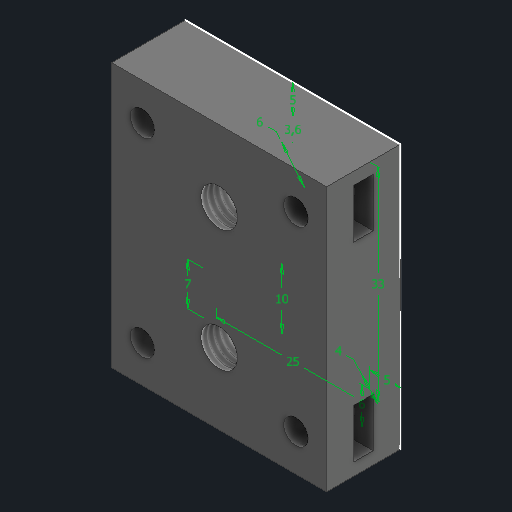
# Autodesk Inventor part: LoadCellBase
Saved by Autodesk Inventor 2027 (Build 310192060, 192F)
## iProperties
Created: 2026-10-06
Part Number: LoadCellBase
Material: Genérico
Document SubType Name: Modeling
Designer: EspacoMaker
Density: 1 g/cm^3
Appearance: Padrão
Author: EspacoMaker
Autodesk Inventor part; units mm, degrees
ref_plane "YZ Plane" through (0, 0, 0) normal (1, 0, 0) x (0, 1, 0)
ref_plane "XZ Plane" through (0, 0, 0) normal (0, 1, 0) x (-1, 0, 0)
ref_plane "XY Plane" through (0, 0, 0) normal (0, 0, 1) x (1, 0, 0)
sketch "EsboçoBase" plane through (0, 0, 0) normal (0, 0, 1) x (1, 0, 0)
  line L0 (-12.5, 16.5) -> (12.5, 16.5) construction
  line L1 (12.5, 16.5) -> (12.5, -16.5) construction
  line L2 (12.5, -16.5) -> (-12.5, -16.5) construction
  line L3 (-12.5, -16.5) -> (-12.5, 16.5) construction
  line L4 (-12.5, 16.5) -> (12.5, -16.5) construction
  line L5 (12.5, 16.5) -> (-12.5, -16.5) construction
  line L6 (0, 16.5) -> (0, -16.5) construction
  line L7 (-12.5, 12.9) -> (12.5, 12.9) construction
  circle A0 centre (0, 9.9) radius 3
  line L8 (-12.5, 0) -> (12.5, 0) construction
  circle A1 centre (0, -9.9) radius 3
  line L9 (17.5, 21.5) -> (-17.5, 21.5)
  line L10 (-17.5, 21.5) -> (-17.5, -21.5)
  line L11 (-17.5, -21.5) -> (17.5, -21.5)
  line L12 (17.5, -21.5) -> (17.5, 21.5)
  line L13 (-2.8868, -4.9) -> (2.8868, -4.9)
  line L14 (2.8868, -4.9) -> (5.7735, -9.9)
  line L15 (5.7735, -9.9) -> (2.8868, -14.9)
  line L16 (2.8868, -14.9) -> (-2.8868, -14.9)
  line L17 (-2.8868, -14.9) -> (-5.7735, -9.9)
  line L18 (-5.7735, -9.9) -> (-2.8868, -4.9)
  line L19 (-2.8868, 4.9) -> (2.8868, 4.9)
  line L20 (2.8868, 4.9) -> (5.7735, 9.9)
  line L21 (5.7735, 9.9) -> (2.8868, 14.9)
  line L22 (2.8868, 14.9) -> (-2.8868, 14.9)
  line L23 (-2.8868, 14.9) -> (-5.7735, 9.9)
  line L24 (-5.7735, 9.9) -> (-2.8868, 4.9)
  circle A2 centre (12.5, -15.5) radius 2
  circle A3 centre (12.5, 15.5) radius 2
  circle A4 centre (-12.5, -15.5) radius 2
  circle A5 centre (-12.5, 15.5) radius 2
  line L25 (-14.5207, -12) -> (-10.4793, -12)
  line L26 (-10.4793, -12) -> (-8.4585, -15.5)
  line L27 (-8.4585, -15.5) -> (-10.4793, -19)
  line L28 (-10.4793, -19) -> (-14.5207, -19)
  line L29 (-14.5207, -19) -> (-16.5415, -15.5)
  line L30 (-16.5415, -15.5) -> (-14.5207, -12)
  point P0 (0, 0)
  point P1 (0, -9.9)
  dimension "d0" = 25
  dimension "d1" = 33
  dimension "d2" = 3.6
  dimension "d3" = 6
  dimension "d4" = 5
  dimension "d22" = 10
  dimension "d29" = 4
  dimension "d30" = 6
  dimension "d31" = 5
  dimension "d38" = 7
  constraints: 62 end point, 10 symmetric about line, 6 centre point, 6 midpoint, 5 parallel, 3 horizontal, 2 coincident, 2 perpendicular, 1 point on line, 1 tangent, 33 other
  measures "d0" distance of L1.end L2.end
  measures "d1" distance of L0.end L1.end
  measures "d2" distance between parallel lines of L0 L7
  measures "d3" diameter of A0
  measures "d4" distance between parallel lines of L0 L9
  measures "d22" distance between parallel lines of L13 L16
  measures "d29" diameter of A2
  measures "d30" distance from line of A2.centre L11
  measures "d31" distance from line of L12 A2.centre
  measures "d38" distance between parallel lines of L25 L28
extrude "Adaptador" add sketch "EsboçoBase" along normal blind 12 contours A0 | A1 | L12 L11 L10 L9 | L13 L14 L15 L16 L17 L18 | L24 L23 L22 L21 L20 L19 | A2 | A3 | A4 | A5 | L25 L26 L27 L28 L29 L30
extrude "Furos" cut sketch "EsboçoBase" along normal blind 15 contours A0 | A1
thread "Thread1" size "M6x1" class "6H" standard "ANSI Metric M Profile" full length
thread "Thread2" size "M6x1" class "6H" standard "ANSI Metric M Profile" full length
sketch "Sketch5" plane through (-17.5, -21.5, 0) normal (-1, 0, 0) x (0, 0, 1)
  point P0 (0, 21.5)
extrude "Extrusion5" cut sketch "EsboçoBase" along normal blind 2 contours L13 L14 L15 L16 L17 L18 | L24 L23 L22 L21 L20 L19
sketch "PorcasLaterais" plane through (-17.5, -21.5, 0) normal (-1, 0, 0) x (0, 0, 1)
  line L0 (4.4, 2) -> (7.6, 2)
  line L1 (7.6, 2) -> (7.6, 10)
  line L2 (7.6, 10) -> (4.4, 10)
  line L3 (4.4, 10) -> (4.4, 2)
  line L4 (0, 0) -> (12, 0) projected
  line L5 (0, 43) -> (0, 0) projected
  line L6 (4.4, 6) -> (7.6, 6) construction
  line L7 (6, 2) -> (6, 10) construction
  line L8 (6, 0) -> (6, 43) construction
  line L9 (0, 6) -> (12, 6) construction
  line L10 (12, 43) -> (12, 0) projected
  point P0 (0, 21.5)
  dimension "d32" = 3.2
  dimension "d33" = 8
  dimension "d37" = 6
  constraints: 16 end point, 5 midpoint, 2 collinear, 2 horizontal, 2 parallel, 2 point on line, 1 perpendicular, 1 vertical
  measures "d32" distance of L2.end L1.end
  measures "d33" distance of L1.end L0.end
  measures "d37" distance between parallel lines of L9 L4
extrude "Extrusion6" cut sketch "PorcasLaterais" against normal blind 9.5
sketch "Sketch7" plane through (-17.5, -19.5, 7.6) normal (0, 0, -1) x (-1, 0, 0)
  line L0 (-9.0415, 4) -> (-7.0207, 0.5) projected
  line L1 (-7.0207, 7.5) -> (-9.0415, 4) projected
  line L2 (-2.9793, 7.5) -> (-7.0207, 7.5) projected
  line L3 (-0.9585, 4) -> (-2.9793, 7.5) projected
  line L4 (-2.9793, 0.5) -> (-0.9585, 4) projected
  line L5 (-7.0207, 0.5) -> (-2.9793, 0.5) projected
  point P0 (-17.5, 19.5)
extrude "Extrusion7" cut sketch "Sketch7" against normal blind 1
extrude "Extrusion8" cut sketch "EsboçoBase" along normal blind 12 contours A2 | A3 | A4 | A5
mirror "Mirror1" about plane through (0, 0, 0) normal (1, 0, 0) of "Extrusion6", "Extrusion7"
mirror "Mirror2" about plane through (0, 0, 0) normal (0, 1, 0) of "Extrusion7", "Extrusion6", "Mirror1"
